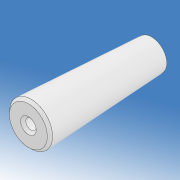
# Autodesk Inventor part: NASA-20-HUB-SPK-01-REV1-PATTERN-RISER
Saved by Autodesk Inventor 2020 (Build 240168000, 168)
## iProperties
Created: 2020-01-06
Part Number: NASA-20-HUB-SPK-01-REV1-PATTERN-RISER
Material: ABS Plastic
Document SubType Name: Modeling
Designer: Rick Szalay
Density: 1.06 g/cm^3
Appearance: Smooth - White
Author: Rick Szalay
Autodesk Inventor part; units mm, degrees
ref_plane "YZ Plane" through (0, 0, 0) normal (1, 0, 0) x (0, 1, 0)
ref_plane "XZ Plane" through (0, 0, 0) normal (0, 1, 0) x (-1, 0, 0)
ref_plane "XY Plane" through (0, 0, 0) normal (0, 0, 1) x (1, 0, 0)
sketch "Sketch1" plane through (0, 0, 0) normal (0, 0, 1) x (1, 0, 0)
  circle A0 centre (101.6, 0) radius 6.35 construction
  circle A1 centre (101.6, 0) radius 8.89
  point P0 (0, 0)
  dimension "d0" = 17.78
  constraints: 1 centre point, 1 coincident
  measures "d0" diameter of A1
extrude "Extrusion1" add sketch "Sketch1" along normal blind 72.0725
draft "FaceDraft1" angle 3 pull direction (0, 0, -1) fixed plane through (104.4772, 2.0451, 0) normal (0, 0, -1) faces at (110.4612, -0.7153, 48.0483)
sketch "Sketch2" plane through (101.6, 0, 0) normal (0, 0, -1) x (-1, 0, 0)
  circle A0 centre (0, 0) radius 6.6675
  point P0 (101.6, 0)
  dimension "d4" = 13.335
  constraints: 1 centre point
  measures "d4" diameter of A0
extrude "Extrusion2" cut sketch "Sketch2" against normal blind 6.985
draft "FaceDraft2" angle 5 pull direction (0, 0, -1) fixed plane through (109.5985, -1.2411, 0) normal (0, 0, -1) faces at (95.0188, -1.0695, 4.6567)
sketch "Sketch3" plane through (101.6, 0, 72.0725) normal (0, 0, 1) x (1, 0, 0)
  point P0 (-101.6, 0)
  point P1 (0, 0)
hole "Hole1" at (101.6, 0, 72.0725) direction (0, 0, -1) diameter 6.096 end through all
chamfer "Chamfer1" distance 1.5875 angle 45 1 edges at (88.9328, 0, 72.0725)
chamfer "Chamfer2" distance 1.524 angle 45 1 edges at (101.6, 3.048, 72.0725)
body "Solid1"
